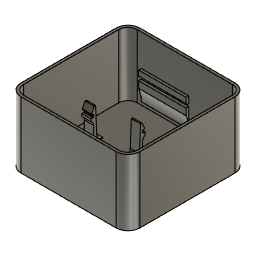
FlameSenderCover (Autodesk Fusion 360 design; units mm, degrees)
part number: 2025-06-28-19-30-18-940
part number: 2025-06-28-21-40-59-564
Autodesk Fusion 360 part; units mm, degrees
sketch "Sketch1" plane through (0, 0, 0) normal (0, 0, 1) x (1, 0, 0)
  line L0 (0, 0) -> (90, 0)
  line L1 (90, 0) -> (90, 90)
  line L2 (90, 90) -> (0, 90)
  line L3 (0, 90) -> (0, 0)
  dimension "d2" = 90
  dimension "d3" = 90
  constraint horizontal L0
  constraint vertical L1
  constraint horizontal L2
  constraint vertical L3
  constraint coincident L0.start L3.end
  measures "d2" distance of L0.start L0.end
  measures "d3" distance of L0.end L1.end
extrude "Extrude1" add sketch "Sketch1" along normal blind 50 makes body 1
fillet "Fillet1" radius 9 4 edges at (0, 0, 25) (90, 0, 25) (90, 90, 25) (0, 90, 25) on bodies 1
shell "Shell1" thickness 2 removed faces 1 at (57, 36, 50) on bodies 1
ref_plane "WorkPlane1" through (47, 45, 26) normal (1, 0, 0) x (0, 1, 0)
ref_plane "WorkPlane2" through (12, 45, 26) normal (1, 0, 0) x (0, 1, 0)
sketch "Sketch2" plane through (12, 0, 0) normal (1, 0, 0) x (0, 1, 0)
  line L0 (2, 26) -> (4, 26)
  line L1 (4, 26) -> (4, 22)
  line L2 (3, 21) -> (2, 21)
  line L3 (2, 21) -> (2, 26)
  line L4 (4, 19) -> (4, 14)
  line L5 (2, 14) -> (2, 19)
  line L6 (4, 14) -> (2, 14)
  line L7 (2, 19) -> (4, 19)
  line L8 (2, 50) -> (2, 2)
  arc A0 (3, 21) -> (4, 22) centre (3, 22) ccw
  line L9 (4, 14) -> (2, 14)
  line L10 (2, 14) -> (4, 14)
  point P0 (4, 21)
  dimension "d13" = 2
  dimension "d14" = 2
  dimension "d15" = 17
  dimension "d16" = 5
  dimension "d17" = 1
  constraint perpendicular L0 L1
  constraint perpendicular L1 L2
  constraint parallel L1 L3
  constraint perpendicular L4 L7
  constraint perpendicular L4 L6
  constraint parallel L4 L5
  constraint equal L0 L7
  constraint coincident L0.start L8
  constraint coincident L2.end L8
  constraint coincident L5.end L8
  constraint coincident L5.start L8
  constraint coincident P0 L2
  constraint coincident P0 L1
  constraint tangent L2 A0
  constraint tangent L1 A0
  constraint equal L3 L5
  measures "d13" distance of L0.start L0.end
  measures "d14" distance of L2 L7
  measures "d15" distance of L5.end L8.end
  measures "d16" distance of L0.end P0
  measures "d17" radius of A0
ref_plane "WorkPlane3" through (78, 45, 26) normal (-1, 0, 0) x (0, -1, 0)
extrude "Extrude2" add sketch "Sketch2" along normal up to surface (66 mm away) bodies 1
fillet "Fillet2" radius 25 1 edges at (45, 2, 14) on bodies 1
sketch "Sketch3" plane through (12, 0, 0) normal (1, 0, 0) x (0, 1, 0)
  line L0 (43.9533, 21) -> (44.5, 21)
  line L1 (45, 20.5) -> (45, 19.5)
  line L2 (44.5, 19) -> (43, 19)
  line L3 (43, 19) -> (43, 17)
  line L4 (43, 17) -> (44.1213, 15.8787)
  line L5 (45, 13.7574) -> (45, 6.9996)
  line L6 (43.5002, 21.7113) -> (45.5, 26)
  line L7 (45.5, 26) -> (46.5, 26)
  line L8 (46.5, 26) -> (47.5, 2)
  line L9 (2, 26) -> (4, 26)
  line L10 (2, 19) -> (4, 19)
  line L11 (3, 21) -> (2, 21)
  arc A0 (40.0607, 2) -> (45, 6.9996) centre (40, 6.9996) ccw
  line L12 (81, 2) -> (9, 2)
  line L13 (2, 2) -> (2, 50)
  line L14 (40.0607, 2) -> (47.5, 2)
  arc A1 (43.5002, 21.7113) -> (43.9533, 21) centre (43.9533, 21.5) ccw
  arc A2 (45, 20.5) -> (44.5, 21) centre (44.5, 20.5) ccw
  arc A3 (44.5, 19) -> (45, 19.5) centre (44.5, 19.5) ccw
  arc A4 (45, 13.7574) -> (44.1213, 15.8787) centre (42, 13.7574) ccw
  point P0 (45, 19)
  point P1 (45, 15)
  dimension "d23" = 5
  dimension "d24" = 65
  dimension "d25" = 2
  dimension "d26" = 13
  dimension "d28" = 2
  dimension "d30" = 43
  dimension "d32" = 45
  dimension "d37" = 1
  dimension "d39" = 0.5
  dimension "d40" = 0.5
  dimension "d41" = 0.5
  dimension "d42" = 3
  constraint horizontal L0
  constraint perpendicular L0 L1
  constraint perpendicular L1 L2
  constraint perpendicular L2 L3
  constraint perpendicular L2 L5
  constraint parallel L0 L7
  constraint collinear L7 L9
  constraint collinear L2 L10
  constraint collinear L0 L11
  constraint tangent L5 A0
  constraint coincident L12 A0.start
  constraint coincident L12 L8.end
  constraint tangent L6 A1
  constraint tangent L0 A1
  constraint tangent L0 A2
  constraint tangent L1 A2
  constraint coincident P0 L1
  constraint coincident P0 L2
  constraint tangent L1 A3
  constraint tangent L2 A3
  constraint coincident P1 L4
  constraint coincident P1 L5
  constraint tangent L4 A4
  constraint tangent L5 A4
  constraint coincident A0.start L14.start
  measures "d23" radius of A0
  measures "d24" angle of L6 L7
  measures "d25" distance of L2.end L3.end
  measures "d26" distance of P1 L12
  measures "d28" distance of P0 L2.end
  measures "d30" distance of L1 L13
  measures "d32" angle of L4 L12
  measures "d37" distance of L6.end L7.end
  measures "d39" radius of A1
  measures "d40" radius of A2
  measures "d41" radius of A3
  measures "d42" radius of A4
extrude "Extrude3" add sketch "Sketch3" along normal blind 7 bodies 1
fillet "Fillet3" radius 5 1 edges at (15.5, 47.5, 2) on bodies 1
fillet "Fillet4" radius 3 2 edges at (19, 46.1784, 2) (12, 46.1784, 2) on bodies 1
pattern_linear "R-Pattern1" count 2 spacing 55 along (1, 0, 0) of "Extrude3", "Fillet3", "Fillet4"
sketch "Sketch4" plane through (12, 0, 0) normal (1, 0, 0) x (0, 1, 0)
  line L0 (86, 14) -> (88, 14)
  line L1 (88, 14) -> (86, 14)
  arc A0 (87, 21) -> (86, 22) centre (87, 22) cw
  line L2 (88, 26) -> (86, 26)
  line L3 (87, 21) -> (88, 21)
  line L4 (86, 19) -> (86, 14)
  line L5 (88, 14) -> (88, 19)
  line L6 (88, 21) -> (88, 26)
  line L7 (86, 14) -> (88, 14)
  line L8 (88, 19) -> (86, 19)
  line L9 (86, 26) -> (86, 22)
  line L10 (88, 2) -> (81, 2)
  line L11 (88, 50) -> (88, 2)
  point P0 (86, 21)
  dimension "d54" = 2
  dimension "d55" = 5
  dimension "d56" = 1
  dimension "d60" = 2
  dimension "d80" = 17
  constraint parallel L6 L9
  constraint perpendicular L4 L8
  constraint perpendicular L0 L4
  constraint parallel L4 L5
  constraint coincident P0 L3
  constraint coincident P0 L9
  constraint tangent A0 L3
  constraint tangent A0 L9
  constraint perpendicular L2 L9
  constraint coincident P0 L4
  constraint equal L5 L6
  constraint coincident L2.start L11
  constraint coincident L3.end L11
  constraint coincident L5.end L11
  constraint coincident L0.end L11
  measures "d54" distance of L3 L8
  measures "d55" distance of P0 L2.end
  measures "d56" radius of A0
  measures "d60" distance of L2.start L2.end
  measures "d80" distance of L8 L10.end
extrude "Extrude4" add sketch "Sketch4" along normal blind 36 bodies 1
fillet "Fillet5" radius 25 1 edges at (30, 88, 14) on bodies 1
ref_plane "WorkPlane4" through (48, 87, 16.5) normal (1, 0, 0) x (0, 0, -1)
sketch "Sketch5" plane through (48, 0, 0) normal (1, 0, 0) x (0, 1, 0)
  line L0 (54.0467, 21) -> (53.5, 21)
  arc A0 (54.4998, 21.7113) -> (54.0467, 21) centre (54.0467, 21.5) cw
  line L1 (53, 13.7574) -> (53, 7)
  line L2 (54.4998, 21.7113) -> (52.5, 26)
  arc A1 (53, 13.7574) -> (53.8787, 15.8787) centre (56, 13.7574) cw
  line L3 (58, 2) -> (50.5, 2)
  arc A2 (53.5, 19) -> (53, 19.5) centre (53.5, 19.5) cw
  arc A3 (58, 2) -> (53, 7) centre (58, 7) cw
  arc A4 (53, 20.5) -> (53.5, 21) centre (53.5, 20.5) cw
  line L4 (51.5, 26) -> (50.5, 2)
  line L5 (55, 19) -> (55, 17)
  line L6 (55, 17) -> (53.8787, 15.8787)
  line L7 (52.5, 26) -> (51.5, 26)
  line L8 (53, 20.5) -> (53, 19.5)
  line L9 (53.5, 19) -> (55, 19)
  line L10 (81, 2) -> (9, 2)
  line L11 (88, 50) -> (88, 2)
  point P0 (53, 19)
  point P1 (53, 15)
  dimension "d64" = 5
  dimension "d65" = 65
  dimension "d66" = 2
  dimension "d68" = 2
  dimension "d70" = 1
  dimension "d71" = 0.5
  dimension "d72" = 0.5
  dimension "d73" = 0.5
  dimension "d74" = 3
  dimension "d75" = 35
  dimension "d81" = 2
  dimension "d82" = 2.5
  dimension "d83" = 24
  dimension "d84" = 11.7574
  dimension "d86" = 30
  dimension "d88" = 7.5
  constraint perpendicular L0 L8
  constraint perpendicular L8 L9
  constraint perpendicular L5 L9
  constraint perpendicular L1 L9
  constraint parallel L0 L7
  constraint tangent L1 A3
  constraint tangent A0 L2
  constraint tangent L0 A0
  constraint tangent L0 A4
  constraint tangent A4 L8
  constraint coincident P0 L8
  constraint coincident P0 L9
  constraint tangent A2 L8
  constraint tangent A2 L9
  constraint coincident P1 L6
  constraint coincident P1 L1
  constraint tangent A1 L6
  constraint tangent L1 A1
  constraint coincident L3.start A3.start
  constraint coincident L3.end L10
  constraint coincident L3.start L10
  measures "d64" radius of A3
  measures "d65" angle of L2 L7
  measures "d66" distance of L5.end L5.start
  measures "d68" distance of L5.start P0
  measures "d70" distance of L2.end L4.start
  measures "d71" radius of A0
  measures "d72" radius of A4
  measures "d73" radius of A2
  measures "d74" radius of A1
  measures "d75" distance of L8 L11
  measures "d81" distance of L0 L9
  measures "d82" distance of L2.end L5
  measures "d83" distance of L7 L10
  measures "d84" distance of A1.centre L10
  measures "d86" distance of L3.start L11
  measures "d88" horizontal distance of A3.centre L3.end
extrude "Extrude5" add sketch "Sketch5" against normal blind 7 bodies 1
fillet "Fillet6" radius 5 1 edges at (44.5, 50.5, 2) on bodies 1
delete_face "DeleteFace1" 1 faces at (21.1477, 47.6694, 2.1236) on bodies 1
delete_face "DeleteFace2" 1 faces at (10.1319, 44.4819, 2.2217) on bodies 1
delete_face "DeleteFace3" 1 faces at (76.1477, 47.6694, 2.1236) on bodies 1
delete_face "DeleteFace4" 1 faces at (64.7671, 44.5135, 2.0997) on bodies 1
copy_body "Body->Comp1" bodies 1 removing the originals makes body 2 in component "Component"
component "Component" placed x (1, 0, 0) y (0, 1, 0) z (0, 0, 1) at (0, 0, 0)
equation "outer_size = 90 mm"
equation "d2 = outer_size"
equation "d3 = outer_size"
equation "outer_radius = 9 mm"
equation "d8 = outer_radius"
equation "wall_thickness = 2 mm"
equation "d10 = wall_thickness"
equation "d11 = outer_size / 2"
